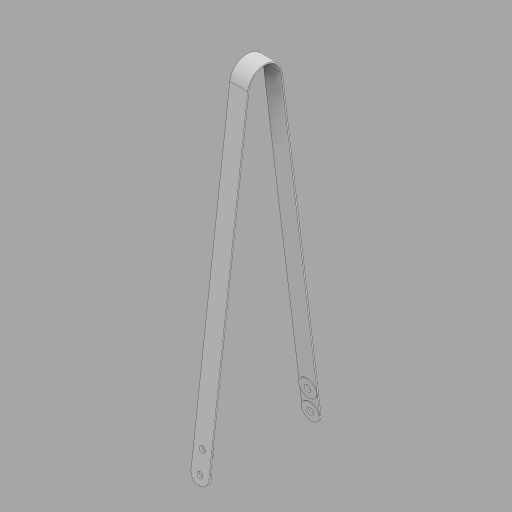
# Autodesk Inventor part: szalag5
Saved by Autodesk Inventor 2023 (Build 270158000, 158)
## iProperties
Created: 2022-11-18
Part Number: szalag5
Material: Generic
Document SubType Name: Modeling
Designer: gd1
Density: 1 g/cm^3
Appearance: Default
Author: gd1
Autodesk Inventor part; units mm, degrees
ref_plane "YZ Plane" through (0, 0, 0) normal (1, 0, 0) x (0, 1, 0)
ref_plane "XZ Plane" through (0, 0, 0) normal (0, 1, 0) x (-1, 0, 0)
ref_plane "XY Plane" through (0, 0, 0) normal (0, 0, 1) x (1, 0, 0)
sketch "Sketch1" plane through (0, 0, 0) normal (1, 0, 0) x (0, 1, 0)
  circle A0 centre (0, 0) radius 14.612
  line L0 (0, 0) -> (-254.37, 0)
  line L1 (0, 0) -> (254.37, 0) construction
  line L2 (-271.87, -50) -> (-236.87, -50)
  line L3 (-236.87, -50) -> (-236.87, 50) construction
  line L4 (-236.87, 50) -> (-271.87, 50)
  line L5 (-271.87, 50) -> (-271.87, -50) construction
  line L6 (-271.87, -50) -> (-236.87, 50) construction
  line L7 (-236.87, -50) -> (-271.87, 50) construction
  line L8 (-271.87, 50) -> (-271.87, 48)
  line L9 (-271.87, 48) -> (1.7754, 14.5037)
  circle A1 centre (0, 0) radius 13.612
  line L10 (-271.87, 48) -> (-271.87, 47)
  line L11 (-271.87, 47) -> (1.6542, 13.5111)
  line L12 (-271.87, -48) -> (1.7754, -14.5037)
  line L13 (-271.87, -47) -> (1.6542, -13.5111)
  line L14 (-271.87, -48) -> (-271.87, -47)
  point P0 (1.6542, -13.5111)
  point P1 (1.7754, -14.5037)
  dimension "d0" = 29.224
  dimension "d6" = 1
  dimension "d1" = 254.37
  dimension "d2" = 180
  dimension "d3" = 35
  dimension "d4" = 100
  dimension "d5" = 2
  dimension "d7" = 1
  constraints: 30 end point, 4 symmetric about line, 3 horizontal, 2 collinear, 2 midpoint, 2 parallel, 2 point on line, 1 coincident, 1 perpendicular, 8 other
  measures "d1" distance of L0.start L0.end
  measures "d2" angle of L0 L1
  measures "d3" distance of L4.end L3.end
  measures "d4" distance of L3.end L2.end
  measures "d5" distance of L4.end L8.end
  measures "d7" distance of L8.end L10.end
extrude "Extrusion1" add sketch "Sketch1" along normal blind 15 contours A0 L13 A1 L11 | A0 L11 L10 L9 | L12 L14 L13 A0
sketch "Sketch2" plane through (15, 1.6542, 13.5111) normal (0, -0.1215273, -0.9925881) x (-1, 0, 0)
  line L0 (15, -275.6882) -> (0, -275.6882) projected
  line L1 (15, -275.6882) -> (0, -275.6882)
  line L2 (0, -275.6882) -> (0, -260.6882)
  line L3 (0, -260.6882) -> (15, -260.6882)
  line L4 (15, -260.6882) -> (15, -275.6882)
  line L5 (15, -0.0004) -> (15, -275.6882) projected
  line L6 (0, -260.6882) -> (15, -260.6882)
  line L7 (15, -260.6882) -> (15, -258.1882)
  line L8 (15, -258.1882) -> (0, -258.1882)
  line L9 (0, -258.1882) -> (0, -260.6882)
  line L10 (15, -258.1882) -> (0, -258.1882)
  line L11 (0, -258.1882) -> (0, -243.1882)
  line L12 (0, -243.1882) -> (15, -243.1882)
  line L13 (15, -243.1882) -> (15, -258.1882)
  circle A0 centre (7.5, -250.6882) radius 7.5
  circle A1 centre (7.5, -268.1882) radius 7.5
  circle A2 centre (7.5, -268.1882) radius 2.3821
  circle A3 centre (7.5, -250.6882) radius 2.3821
  point P0 (15, 0)
  point P1 (15, -268.1882)
  point P2 (7.5, -275.6882)
  point P3 (0, -268.1882)
  point P4 (0, -275.6882)
  dimension "d10" = 15
  dimension "d11" = 15
  dimension "d12" = 2.5
  dimension "d13" = 15
  dimension "d14" = 15
  constraints: 24 end point, 6 parallel, 4 centre point, 3 horizontal, 3 perpendicular, 2 coincident, 1 point on line, 1 tangent
  measures "d10" distance of L2.end L3.end
  measures "d11" distance of L1.end L2.end
  measures "d12" distance of L7.end L6.end
  measures "d13" distance of L11.end L12.end
  measures "d14" distance of L10.end L11.end
extrude "Extrusion2" add sketch "Sketch2" along normal blind 1 contours A1 | A0 | A2 | A3
extrude "Extrusion3" cut sketch "Sketch2" along normal mid plane 2 contours A2 | A3
extrude "Extrusion4" cut sketch "Sketch2" along normal mid plane 2 contours L0 A1 L4 | L0 L2 A1
sketch "Sketch3" plane through (0, -271.87, -47) normal (0, -0.1215273, 0.9925881) x (1, 0, 0)
  line L0 (0, -0.1215) -> (15, -0.1215) projected
  line L1 (0, -0.1215) -> (15, -0.1215)
  line L2 (15, -0.1215) -> (15, 14.8785)
  line L3 (15, 14.8785) -> (0, 14.8785)
  line L4 (0, 14.8785) -> (0, -0.1215)
  line L5 (0, -0.1215) -> (0, 275.5663) projected
  line L6 (15, 14.8785) -> (0, 14.8785)
  line L7 (0, 14.8785) -> (0, 17.3785)
  line L8 (0, 17.3785) -> (15, 17.3785)
  line L9 (15, 17.3785) -> (15, 14.8785)
  line L10 (0, 17.3785) -> (15, 17.3785)
  line L11 (15, 17.3785) -> (15, 33.5951)
  line L12 (15, 33.5951) -> (0, 33.5951)
  line L13 (0, 33.5951) -> (0, 17.3785)
  circle A0 centre (7.5, 7.3785) radius 7.5
  circle A1 centre (7.5, 25.4868) radius 7.5
  circle A2 centre (7.5, 7.3785) radius 2.75
  circle A3 centre (7.5, 25.4868) radius 2.75
  point P0 (0, 275.5667)
  point P1 (15, 7.3785)
  point P2 (7.5, -0.1215)
  point P3 (0, 7.3785)
  dimension "d21" = 15
  dimension "d22" = 15
  dimension "d23" = 2.5
  dimension "d24" = 15
  dimension "d27" = 5.5
  dimension "d28" = 5.5
  constraints: 24 end point, 6 parallel, 4 centre point, 3 horizontal, 3 perpendicular, 2 coincident, 1 point on line, 1 tangent
  measures "d21" distance of L3.end L2.end
  measures "d22" distance of L2.end L1.end
  measures "d23" distance of L6.end L7.end
  measures "d24" distance of L12.end L11.end
  measures "d27" diameter of A2
  measures "d28" diameter of A3
extrude "Extrusion5" add sketch "Sketch3" along normal mid plane 1 contours A0 | A1 | A2 | A3
extrude "Extrusion6" cut sketch "Sketch3" along normal mid plane 2 contours A2 | A3
extrude "Extrusion7" cut sketch "Sketch3" along normal mid plane 2 contours L4 A0 L0 | A0 L2 L0
body "Solid1"
